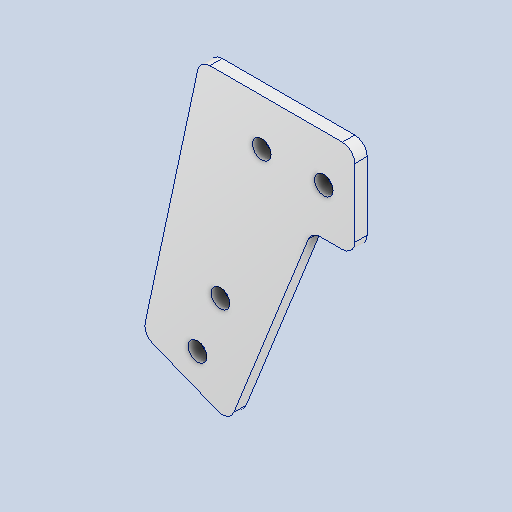
# Autodesk Inventor part: dribl-v4-Plate-2
Saved by Autodesk Inventor 2025.2 (Build 292293000, 293)
## iProperties
Created: 2025-05-12
Part Number: dribl-v4-Plate-2
Material: アルミニウム 6061
Document SubType Name: Modeling
Designer: haruy
Density: 2.7 g/cm^3
Appearance: アルミニウム - フラット
Author: haruy
Autodesk Inventor part; units mm, degrees
ref_plane "YZ Plane" through (0, 0, 0) normal (1, 0, 0) x (0, 1, 0)
ref_plane "XZ Plane" through (0, 0, 0) normal (0, 1, 0) x (-1, 0, 0)
ref_plane "XY Plane" through (0, 0, 0) normal (0, 0, 1) x (1, 0, 0)
derived "dribl-v3-ASP-arm.ipt"
sketch "スケッチ31" plane through (31.5, 52, 25) normal (0, 0, 1) x (1, 0, 0)
  line L0 (-498.5, 298) -> (-124.5, 298) projected
  line L1 (-124.5, 298) -> (-124.5, 283) projected
  line L2 (-124.5, 283) -> (-498.5, 283) projected
  line L3 (-498.5, 283) -> (-498.5, 298) projected
  line L4 (-438.5, 298) -> (-423.5, 298) projected
  line L5 (-488.5, 223) -> (-134.5, 223) projected
  line L6 (-134.5, 223) -> (-134.5, 208) projected
  line L7 (-134.5, 208) -> (-488.5, 208) projected
  line L8 (-488.5, 208) -> (-488.5, 223) projected
  line L9 (-626.9117, 6.1467) -> (-613.3232, -0.2057) projected
  line L10 (-613.3232, -0.2057) -> (-486.2756, 271.5643) projected
  line L11 (-486.2756, 271.5643) -> (-499.8641, 277.9166) projected
  line L12 (-499.8641, 277.9166) -> (-626.9117, 6.1467) projected
  line L13 (-593.8173, -61.3723) -> (-579.8804, -66.9189) projected
  line L14 (-579.8804, -66.9189) -> (-474.4952, 197.8809) projected
  line L15 (-474.4952, 197.8809) -> (-488.432, 203.4275) projected
  line L16 (-488.432, 203.4275) -> (-593.8173, -61.3723) projected
  circle A0 centre (-618, 7.5) radius 1.5 projected
  circle A1 centre (-618, 7.5) radius 1.5 projected
  line L17 (-438.5, -62) -> (-438.5, 298) projected
  circle A2 centre (-585, -59.5) radius 1.5 projected
  circle A3 centre (-585, -59.5) radius 1.5 projected
  line L18 (-184.5, 298) -> (-184.5, -62) projected
  line L19 (-311.5, 298) -> (-311.5, 208) projected
  line L20 (-9.6768, -0.2057) -> (-136.7244, 271.5643) projected
  line L21 (-123.1359, 277.9166) -> (3.9117, 6.1467) projected
  line L22 (-136.7244, 271.5643) -> (-123.1359, 277.9166) projected
  line L23 (3.9117, 6.1467) -> (-9.6768, -0.2057) projected
  circle A4 centre (-5, 7.5) radius 1.5 projected
  line L24 (-29.1827, -61.3723) -> (-43.1196, -66.9189) projected
  line L25 (-134.568, 203.4275) -> (-29.1827, -61.3723) projected
  circle A5 centre (-38, -59.5) radius 1.5 projected
  line L26 (-43.1196, -66.9189) -> (-148.5048, 197.8809) projected
  line L27 (-148.5048, 197.8809) -> (-134.568, 203.4275) projected
  line L28 (-623, -52) -> (-623, 15) projected
  line L29 (-623, -52) -> (-613, -52) projected
  line L30 (-613, -52) -> (-613, -147) projected
  line L31 (-613, -147) -> (-623, -147) projected
  line L32 (-623, -147) -> (-623, -52) projected
  line L33 (-593.8173, -61.3723) -> (-579.8804, -66.9189) projected
  line L34 (-579.8804, -66.9189) -> (-613.16, -150.5399) projected
  line L35 (-613.16, -150.5399) -> (-627.0968, -144.9933) projected
  line L36 (-627.0968, -144.9933) -> (-593.8173, -61.3723) projected
  circle A6 centre (-618, -142.4186) radius 1.5 projected
  line L37 (-590, -37) -> (-590, 15) projected
  line L38 (-590, 15) -> (-580, 15) projected
  line L39 (-580, 15) -> (-580, 83.0909) projected
  line L40 (-580, 83.0909) -> (-590, 83.0909) projected
  line L41 (-590, 83.0909) -> (-590, 15) projected
  circle A7 centre (-585, 78.0909) radius 1.5 projected
  line L42 (-580, -52) -> (-590, -52) projected
  line L43 (-580, -52) -> (-590, -52) projected
  line L44 (-590, -52) -> (-590, -64.9091) projected
  line L45 (-590, -64.9091) -> (-580, -64.9091) projected
  line L46 (-580, -64.9091) -> (-580, -52) projected
  circle A8 centre (-497.3048, 265.6815) radius 1.5 projected
  circle A9 centre (-501.5397, 256.6225) radius 1.5 projected
  circle A10 centre (-488.5, 290.5) radius 1.5 projected
  circle A11 centre (-478.5, 290.5) radius 1.5 projected
  line L47 (-510.4514, 255.2691) -> (-496.8629, 248.9168) projected
  line L48 (-473.5, 298) -> (-473.5, 283) projected
  line L49 (-486.2756, 271.5643) -> (-480.9296, 283) projected
  line L50 (-498.5, 298) -> (-510.4514, 255.2691) projected
  circle A12 centre (-488.8591, 182.0718) radius 1.5 projected
  circle A13 centre (-485.1614, 191.363) radius 1.5 projected
  circle A14 centre (-478.5, 215.5) radius 1.5 projected
  circle A15 centre (-468.5, 215.5) radius 1.5 projected
  line L51 (-463.5, 223) -> (-463.5, 208) projected
  line L52 (-497.6764, 180.1995) -> (-483.7395, 174.6529) projected
  line L53 (-474.4952, 197.8809) -> (-470.468, 208) projected
  line L54 (-488.5, 223) -> (-497.6764, 180.1995) projected
  line L55 (-560, -23.3648) -> (-537, -23.3648) projected
  line L56 (-537, -23.3648) -> (-537, -43.3648) projected
  line L57 (-537, -43.3648) -> (-560, -43.3648) projected
  line L58 (-560, -43.3648) -> (-560, -23.3648) projected
  circle A16 centre (-555, -28.3648) radius 1.6 projected
  line L59 (-548.5, -23.3648) -> (-548.5, -43.3648) projected
  line L60 (-560, -33.3648) -> (-537, -33.3648) projected
  circle A17 centre (-542, -28.3648) radius 1.6 projected
  circle A18 centre (-542, -38.3648) radius 1.6 projected
  circle A19 centre (-555, -38.3648) radius 1.6 projected
  line L61 (-580, 15) -> (-580, -37) projected
  line L62 (-560, -43.3648) -> (-582.6708, -33.3648) projected
  point P0 (-31.5, -52)
  point P1 (-134.5, 215.5)
  point P2 (-582.0234, -31.738)
  point P3 (-583.5, -35.4482)
extrude "押し出し1" add sketch "スケッチ31" along normal blind 2 contours L51 L7 L8 L5 | L8 L7 L53 L15 L16 L54 | L16 L15 L14 L52
fillet "フィレット1" radius 2 6 edges at (-432, 275, 26) (-438.968, 260, 26) (-432, 260, 26) (-452.2395, 226.6529, 26) (-466.1764, 232.1995, 26) (-457, 275, 26)
